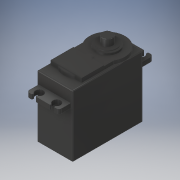
# Autodesk Inventor part: CH_01_0004_servo_update
Saved by Autodesk Inventor 2019 (Build 230136000, 136)
## iProperties
Created: 2022-02-28
Part Number: CH_01_0004_servo_update
Material: Generic
Document SubType Name: Modeling
Designer: Tomasz Krakowski
Density: 1 g/cm^3
Appearance: Ciemnoszara
Author: Tomasz Krakowski
Autodesk Inventor part; units mm, degrees
ref_plane "YZ Plane" through (0, 0, 0) normal (1, 0, 0) x (0, 1, 0)
ref_plane "XZ Plane" through (0, 0, 0) normal (0, 1, 0) x (-1, 0, 0)
ref_plane "XY Plane" through (0, 0, 0) normal (0, 0, 1) x (1, 0, 0)
sketch "Sketch1" plane through (0, 0, 0) normal (0, 1, 0) x (-1, 0, 0)
  line L0 (-10.25, 20.25) -> (10.25, 20.25)
  line L1 (10.25, 20.25) -> (10.25, -20.25)
  line L2 (10.25, -20.25) -> (-10.25, -20.25)
  line L3 (-10.25, -20.25) -> (-10.25, 20.25)
  line L4 (-10.25, 20.25) -> (10.25, -20.25) construction
  line L5 (10.25, 20.25) -> (-10.25, -20.25) construction
  point P0 (0, 0)
  dimension "d0" = 20.5
  dimension "d1" = 40.5
  constraints: 12 end point, 2 midpoint, 2 parallel, 1 horizontal, 1 perpendicular
  measures "d0" distance between parallel lines of L3 L1
  measures "d1" distance between parallel lines of L2 L0
extrude "Extrusion1" add sketch "Sketch1" along normal blind 28.3
sketch "Sketch2" plane through (0, 28.3, 0) normal (0, 1, 0) x (1, 0, 0)
  line L0 (-10.25, -20.25) -> (10.25, -20.25) projected
  line L1 (10.25, -20.25) -> (10.25, 20.25) projected
  line L2 (10.25, 20.25) -> (-10.25, 20.25) projected
  line L3 (-10.25, 20.25) -> (-10.25, -20.25) projected
  line L4 (0, 0) -> (-10.25, 0) construction
  arc A0 (-3.9773, -26.2541) -> (-6.4318, -25.9856) centre (-5, -24.25) ccw
  line L5 (-10.25, -20.25) -> (10.25, -20.25) construction
  line L6 (0, -20.25) -> (0, 0) construction
  line L7 (-6.25, -26.3713) -> (-6.25, -26.75)
  line L8 (-6.75, -27.25) -> (-7.75, -27.25)
  line L9 (-9.25, -25.75) -> (-9.25, -20.25)
  arc A1 (-9.25, -25.75) -> (-7.75, -27.25) centre (-7.75, -25.75) ccw
  line L10 (-4.25, -26.6995) -> (-4.25, -26.75)
  line L11 (-3.75, -27.25) -> (0, -27.25)
  line L12 (0, -27.25) -> (0, -20.25) construction
  arc A2 (-6.75, -27.25) -> (-6.25, -26.75) centre (-6.75, -26.75) ccw
  arc A3 (-4.25, -26.75) -> (-3.75, -27.25) centre (-3.75, -26.75) ccw
  arc A4 (-3.9773, -26.2541) -> (-4.25, -26.6995) centre (-3.75, -26.6995) ccw
  arc A5 (-6.25, -26.3713) -> (-6.4318, -25.9856) centre (-6.75, -26.3713) ccw
  arc A6 (6.4318, -25.9856) -> (3.9773, -26.2541) centre (5, -24.25) ccw
  line L13 (6.25, -26.3713) -> (6.25, -26.75)
  line L14 (6.75, -27.25) -> (7.75, -27.25)
  line L15 (9.25, -25.75) -> (9.25, -20.25)
  arc A7 (7.75, -27.25) -> (9.25, -25.75) centre (7.75, -25.75) ccw
  line L16 (4.25, -26.6995) -> (4.25, -26.75)
  line L17 (3.75, -27.25) -> (0, -27.25)
  arc A8 (6.25, -26.75) -> (6.75, -27.25) centre (6.75, -26.75) ccw
  arc A9 (3.75, -27.25) -> (4.25, -26.75) centre (3.75, -26.75) ccw
  arc A10 (4.25, -26.6995) -> (3.9773, -26.2541) centre (3.75, -26.6995) ccw
  arc A11 (6.4318, -25.9856) -> (6.25, -26.3713) centre (6.75, -26.3713) ccw
  arc A12 (-6.4318, 25.9856) -> (-3.9773, 26.2541) centre (-5, 24.25) ccw
  line L18 (-6.25, 26.3713) -> (-6.25, 26.75)
  line L19 (-6.75, 27.25) -> (-7.75, 27.25)
  line L20 (-9.25, 25.75) -> (-9.25, 20.25)
  arc A13 (-7.75, 27.25) -> (-9.25, 25.75) centre (-7.75, 25.75) ccw
  line L21 (-4.25, 26.6995) -> (-4.25, 26.75)
  line L22 (-3.75, 27.25) -> (0, 27.25)
  line L23 (0, 27.25) -> (0, 20.25) construction
  arc A14 (-6.25, 26.75) -> (-6.75, 27.25) centre (-6.75, 26.75) ccw
  arc A15 (-3.75, 27.25) -> (-4.25, 26.75) centre (-3.75, 26.75) ccw
  arc A16 (-4.25, 26.6995) -> (-3.9773, 26.2541) centre (-3.75, 26.6995) ccw
  arc A17 (-6.4318, 25.9856) -> (-6.25, 26.3713) centre (-6.75, 26.3713) ccw
  arc A18 (9.25, 25.75) -> (7.75, 27.25) centre (7.75, 25.75) ccw
  line L24 (4.25, 26.6995) -> (4.25, 26.75)
  arc A19 (3.9773, 26.2541) -> (4.25, 26.6995) centre (3.75, 26.6995) ccw
  arc A20 (4.25, 26.75) -> (3.75, 27.25) centre (3.75, 26.75) ccw
  arc A21 (3.9773, 26.2541) -> (6.4318, 25.9856) centre (5, 24.25) ccw
  line L25 (9.25, 25.75) -> (9.25, 20.25)
  line L26 (3.75, 27.25) -> (0, 27.25)
  line L27 (6.25, 26.3713) -> (6.25, 26.75)
  line L28 (6.75, 27.25) -> (7.75, 27.25)
  arc A22 (6.75, 27.25) -> (6.25, 26.75) centre (6.75, 26.75) ccw
  arc A23 (6.25, 26.3713) -> (6.4318, 25.9856) centre (6.75, 26.3713) ccw
  line L29 (-9.25, -20.25) -> (9.25, -20.25)
  line L30 (-9.25, 20.25) -> (9.25, 20.25)
  line L31 (10.25, 20.25) -> (-10.25, 20.25) projected
  point P0 (-6.25, -26.1208)
  point P1 (-4.25, -26.3713)
  point P2 (6.25, -26.1208)
  point P3 (4.25, -26.3713)
  point P4 (-6.25, 26.1208)
  point P5 (-4.25, 26.3713)
  point P6 (4.25, 26.3713)
  point P7 (6.25, 26.1208)
  dimension "d4" = 1.5
  dimension "d5" = 7
  dimension "d6" = 4
  dimension "d7" = 4.5
  dimension "d8" = 2
  dimension "d9" = 3
  dimension "d10" = 1
  dimension "d11" = 2
  dimension "d12" = 0.5
  constraints: 59 symmetric about line, 56 point on circle, 52 end point, 24 centre point, 10 tangent, 9 point on line, 4 collinear, 4 perpendicular, 3 equal radius, 2 midpoint, 2 vertical, 18 other
  measures "d4" radius of A1
  measures "d5" distance from line of L8 L9.end
  measures "d6" vertical distance of A0.centre L9.end
  measures "d7" diameter of A0
  measures "d8" distance edge to line of A0 L9
  measures "d9" distance between parallel lines of L9 L7
  measures "d10" distance between parallel lines of L3 L9
  measures "d11" distance between parallel lines of L7 L10
  measures "d12" radius of A2
extrude "Extrusion2" add sketch "Sketch2" along normal blind 2.5
sketch "Sketch3" plane through (0, 30.8, 0) normal (0, 1, 0) x (1, 0, 0)
  line L0 (-9.25, 20.25) -> (-10.25, 20.25) projected
  line L1 (10.25, -20.25) -> (-10.25, -20.25)
  line L2 (-10.25, -20.25) -> (-10.25, 20.25)
  line L3 (-10.25, 20.25) -> (10.25, 20.25)
  line L4 (10.25, 20.25) -> (10.25, -20.25)
  line L5 (10.25, -20.25) -> (-10.25, 20.25) construction
  line L6 (-10.25, -20.25) -> (10.25, 20.25) construction
  point P0 (0, 0)
  constraints: 12 end point, 2 midpoint, 2 parallel, 1 horizontal, 1 perpendicular
extrude "Extrusion3" add sketch "Sketch3" along normal blind 6.6
sketch "Sketch4" plane through (0, 37.4, 0) normal (0, 1, 0) x (1, 0, 0)
  circle A0 centre (0, 10) radius 10.25
  line L0 (0, 0) -> (0, 10) construction
  line L1 (-10.25, 20.25) -> (-10.25, -20.25) construction
  line L2 (10.25, 20.25) -> (-10.25, 20.25) construction
  line L3 (10.25, -20.25) -> (10.25, 20.25) construction
  line L4 (-8.9, 4.9155) -> (-8.9, -13.75)
  line L5 (-8.9, -13.75) -> (-4.9, -13.75)
  line L6 (0, 0) -> (0, -15.0328) construction
  line L7 (0, 10) -> (0, 20.25) construction
  arc A1 (-4.9, -13.75) -> (0, -15.0328) centre (0, -5.0328) ccw
  line L8 (8.9, 4.9155) -> (8.9, -13.75)
  line L9 (8.9, -13.75) -> (4.9, -13.75)
  arc A2 (0, -15.0328) -> (4.9, -13.75) centre (0, -5.0328) ccw
  arc A3 (-8.9, 4.9155) -> (8.9, 4.9155) centre (0, 10) ccw
  arc A4 (3.9773, 26.2541) -> (6.4318, 25.9856) centre (5, 24.25) ccw construction
  dimension "d19" = 8.9
  dimension "d20" = 34
  dimension "d23" = 10
  dimension "d24" = 4
  dimension "d53" = 14.25
  constraints: 15 end point, 6 point on circle, 3 centre point, 3 symmetric about line, 3 vertical, 1 coincident, 1 collinear, 1 horizontal, 1 midpoint, 1 perpendicular, 1 point on line, 4 other
  measures "d19" distance between parallel lines of L4 L6
  measures "d20" distance from line of L5 L7.end
  measures "d23" radius of A1
  measures "d24" distance of L4.end L5.end
  measures "d53" vertical distance of A4.centre L0.end
extrude "Extrusion4" add sketch "Sketch4" along normal blind 2
sketch "Sketch5" plane through (0, 39.4, 0) normal (0, 1, 0) x (1, 0, 0)
  line L0 (-4.9, -13.75) -> (-8.9, -13.75) projected
  line L1 (-8.9, -13.75) -> (8.9, -13.75)
  line L2 (8.9, -13.75) -> (8.9, -0.75)
  line L3 (-8.9, -0.75) -> (-8.9, -13.75)
  line L4 (8.9, -13.75) -> (8.9, 4.9155) construction
  arc A0 (2, -0.75) -> (-2, -0.75) centre (0, -0.75) ccw
  line L5 (8.9, -0.75) -> (2, -0.75)
  line L6 (-2, -0.75) -> (-8.9, -0.75)
  line L7 (0, -0.75) -> (0, 0) construction
  dimension "d26" = 4
  dimension "d27" = 13
  constraints: 12 end point, 3 parallel, 2 collinear, 2 point on circle, 1 centre point, 1 horizontal, 1 horizontal alignment, 1 perpendicular, 1 vertical
  measures "d26" diameter of A0
  measures "d27" distance between parallel lines of L1 L6
extrude "Extrusion5" add sketch "Sketch5" along normal blind 0.5
sketch "Sketch6" plane through (0, 39.4, 0) normal (0, 1, 0) x (1, 0, 0)
  arc A0 (8.9, 4.9155) -> (-8.9, 4.9155) centre (0, 10) ccw construction
  circle A1 centre (0, 10) radius 6.5
  point P0 (0, 0)
  dimension "d30" = 13
  constraints: 1 centre point, 1 coincident
  measures "d30" diameter of A1
extrude "Extrusion6" add sketch "Sketch6" along normal blind 1.25
sketch "Sketch7" plane through (0, 40.65, -10) normal (0, 1, 0) x (1, 0, 0)
  circle A0 centre (0, 0) radius 6.5 construction
  circle A1 centre (0, 0) radius 5.375
  point P0 (0, -10)
  dimension "d33" = 10.75
  constraints: 1 centre point, 1 coincident
  measures "d33" diameter of A1
extrude "Extrusion7" add sketch "Sketch7" along normal blind 0.5
sketch "Sketch8" plane through (0, 41.15, -10) normal (0, 1, 0) x (1, 0, 0)
  circle A0 centre (0, 0) radius 5.375 construction
  circle A1 centre (0, 0) radius 3
  point P0 (0, -10)
  dimension "d36" = 6
  constraints: 1 centre point, 1 coincident
  measures "d36" diameter of A1
extrude "Extrusion8" add sketch "Sketch8" along normal blind 4
chamfer "Chamfer1" distance 0.25 angle 45 1 edges at (-3, 45.15, -10)
sketch "Sketch9" plane through (10.25, 0, -20.25) normal (0, 0, -1) x (-1, 0, 0)
  line L0 (7.5, 3) -> (13, 3)
  line L1 (13.5, 3.5) -> (13.5, 5)
  line L2 (13, 5.5) -> (7.5, 5.5)
  line L3 (7, 5) -> (7, 3.5)
  line L4 (7, 3) -> (13.5, 5.5) construction
  line L5 (13.5, 3) -> (7, 5.5) construction
  line L6 (10.25, 4.25) -> (10.25, 0) construction
  line L7 (0, 0) -> (20.5, 0) construction
  arc A0 (7.5, 5.5) -> (7, 5) centre (7.5, 5) ccw
  arc A1 (7, 3.5) -> (7.5, 3) centre (7.5, 3.5) ccw
  arc A2 (13.5, 5) -> (13, 5.5) centre (13, 5) ccw
  arc A3 (13, 3) -> (13.5, 3.5) centre (13, 3.5) ccw
  dimension "d42" = 6.5
  dimension "d43" = 2.5
  dimension "d44" = 3
  dimension "d45" = 0.5
  dimension "d46" = 0.5
  constraints: 14 end point, 8 point on circle, 8 point on line, 8 tangent, 4 centre point, 2 equal radius, 2 midpoint, 2 parallel, 2 perpendicular, 1 horizontal
  measures "d42" distance between parallel lines of L1 L3
  measures "d43" distance between parallel lines of L0 L2
  measures "d44" distance between parallel lines of L7 L0
  measures "d45" radius of A0
  measures "d46" radius of A1
extrude "Extrusion9" add sketch "Sketch9" along normal blind 3
chamfer "Chamfer2" distance 2 angle 45 4 edges at (0, 0, -20.25) (10.25, 0, 0) (-10.25, 0, 0) (0, 0, 20.25)
fillet "Fillet1" radius 0.5 11 edges at (-10.25, 19.7, -20.25) (10.25, 19.7, -20.25) (-10.25, 19.7, 20.25) (10.25, 19.7, 20.25) (-10.25, 37.4, -15.125) (-5.125, 37.4, -20.25) (5.125, 37.4, -20.25) (-10.25, 37.4, 5.125) (0, 37.4, 20.25) (10.25, 37.4, 5.125) (10.25, 37.4, -15.125)
body "Solid1"
